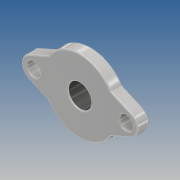
# Autodesk Inventor part: bloklager
Saved by Autodesk Inventor 2018 (Build 220112000, 112)
## iProperties
Created: 2018-10-31
Part Number: bloklager
Material: Aluminum 6061
Document SubType Name: Modeling
Designer: Svend
Density: 2.7 g/cm^3
Appearance: Aluminum - Polished
Author: Svend
Autodesk Inventor part; units mm, degrees
ref_plane "YZ Plane" through (0, 0, 0) normal (1, 0, 0) x (0, 1, 0)
ref_plane "XZ Plane" through (0, 0, 0) normal (0, 1, 0) x (-1, 0, 0)
ref_plane "XY Plane" through (0, 0, 0) normal (0, 0, 1) x (1, 0, 0)
sketch "Sketch1" plane through (0, 0, 0) normal (0, 1, 0) x (-1, 0, 0)
  circle A0 centre (24, 0) radius 3.5
  circle A1 centre (-24, 0) radius 3.5
  arc A2 (-26.4134, 5.4932) -> (-26.4134, -5.4932) centre (-24, 0) ccw
  arc A3 (26.4134, -5.4932) -> (26.4134, 5.4932) centre (24, 0) ccw
  line L0 (26.4134, 5.4932) -> (16.1555, 10)
  line L1 (26.4134, -5.4932) -> (16.1555, -10)
  line L2 (-26.4134, 5.4932) -> (-16.1555, 10)
  line L3 (-26.4134, -5.4932) -> (-16.1555, -10)
  arc A4 (16.1555, 10) -> (-16.1555, 10) centre (0, 0) ccw
  arc A5 (-16.1555, -10) -> (16.1555, -10) centre (0, 0) ccw
  circle A6 centre (0, 0) radius 6
  dimension "d1" = 7
  dimension "d2" = 7
  dimension "d3" = 48
  dimension "d4" = 24
  dimension "d5" = 12
  dimension "d6" = 12
  dimension "d7" = 20
  dimension "d8" = 20
  dimension "d9" = 19
  dimension "d10" = 19
  dimension "d11" = 12
  constraints: 8 end point, 8 point on circle, 7 centre point, 4 coincident, 4 tangent, 2 equal length, 2 horizontal alignment
  measures "d1" diameter of A0
  measures "d2" diameter of A1
  measures "d3" distance of A1.centre A0.centre
  measures "d4" distance of A1.centre A4.centre
  measures "d5" diameter of A2
  measures "d6" diameter of A3
  measures "d7" distance of L1.end L0.end
  measures "d8" distance of L2.end L3.end
  measures "d9" radius of A4
  measures "d10" radius of A5
  measures "d11" diameter of A6
extrude "Extrusion1" add sketch "Sketch1" along normal blind 6
sketch "Sketch2" plane through (0, 6, 0) normal (0, 1, 0) x (1, 0, 0)
  circle A0 centre (0, 0) radius 7.5
  circle A1 centre (0, 0) radius 6
  dimension "d14" = 15
  constraints: 2 centre point, 2 coincident
  measures "d14" diameter of A0
extrude "Extrusion2" add sketch "Sketch2" along normal blind 5
fillet "Fillet1" radius 0.5 23 edges at (-21.2845, 0, 7.7466) (-21.2845, 6, 7.7466) (0, 0, 19) (0, 6, 19) (-30, 0, 0) (-30, 6, 0) (21.2845, 0, 7.7466) (-21.2845, 0, -7.7466) (30, 0, 0) (0, 0, -19) (21.2845, 0, -7.7466) (27.5, 0, 0) (6, 0, 0) (-20.5, 0, 0) (21.2845, 6, 7.7466) (-21.2845, 6, -7.7466) (30, 6, 0) (0, 6, -19) (21.2845, 6, -7.7466) (27.5, 6, 0) (-20.5, 6, 0) (-6, 11, 0) (-7.5, 11, 0)
fillet "Fillet1" radius 0.1 5 edges at (-16.1555, 3, 10) (16.1555, 3, 10) (-7.5, 6, 0) (-16.1555, 3, -10) (16.1555, 3, -10)
equation "\"d4\" = 0.5 * d3"
equation "\"d8\" = d7"
equation "\"d10\" = d9"
body "Solid1"
